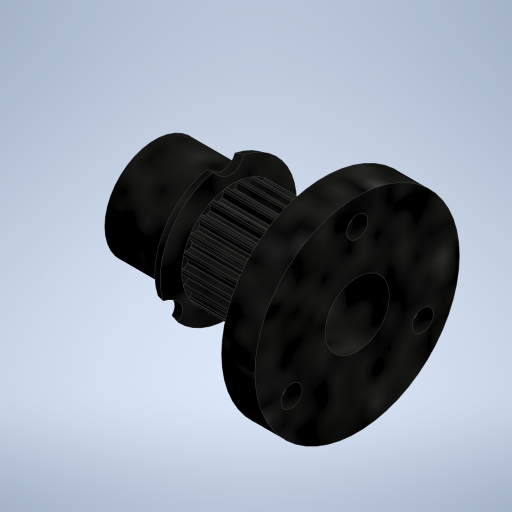
# Autodesk Inventor part: HTPA22S2M100-A-V4-Z6-J3.0_a
Saved by Autodesk Inventor 2024 (Build 280153000, 153)
## iProperties
Category: PARTsolutions
Company: MISUMI
Created: 2025-03-04
Part Number: HTPA22S2M100-A-V4-Z6-J3.0_a
Material: ABS プラスチック
Catalog Web Link: www.cadenas.de
Description: HTPA_ _S2M040, HTPA_ _S2M060, HTPA_ _S2M100, HTPB_ _S2M040, HTPB_ _S2M060, HTPB_ _S2M100, HTPK_ _S2M040, HTPK_ _S2M060, HTPK_ _S2M100, HTPN_ _S2M040, HTPN_ _S2M060, HTPN_ _S2M100, HTPT_ _S2M040, HTPT_ _S2M060, HTPM_ _S2M040, HTPM_ _S2M060, HTPP_ _S2M040, HTPP_ _S2M060, HTPS_ _S2M040, HTPS_ _S2M060, HTPS_ _S2M100_a-High Torque Timing Pulleys S2M Type
Vendor: MISUMI
Document SubType Name: Modeling
Designer: psAdmin
Manufacturer: MISUMI
Mass: 1.84697 g
Surface Area: 17.6348 cm^2
Volume: 1.84697 cm^3
Density: 1.06 g/cm^3
Appearance: 滑らか - 黒
PSOL_IDENT_0: {$CADENAS_DATA/23d-libs/misumi/metric/51_timing_pulleys/htpm_s2m/htpa_s2m.prj},750 {VTYP=3D},{NB=HTP
PSOL_IDENT_1: A22S2M100-A-V4-Z6-J3.0_a},{LINA=HTPA22S2M100-A-V4-Z6-J3.0},{NN=HTPA_ _S2M040, HTPA_ _S2M060, HTPA_ _
PSOL_IDENT_2: S2M100, HTPB_ _S2M040, HTPB_ _S2M060, HTPB_ _S2M100, HTPK_ _S2M040, HTPK_ _S2M060, HTPK_ _S2M100, HT
PSOL_IDENT_3: PN_ _S2M040, HTPN_ _S2M060, HTPN_ _S2M100, HTPT_ _S2M040, HTPT_ _S2M060, HTPM_ _S2M040, HTPM_ _S2M06
PSOL_IDENT_4: 0, HTPP_ _S2M040, HTPP_ _S2M060, HTPS_ _S2M040, HTPS_ _S2M060, HTPS_ _S2M100_a},{DATE=29.05.2023 09:
PSOL_IDENT_5: 16:33},{GEOMDATE=11.01.2023 01:57:31},{VERSION=},{LINEID=70},{WBVAR=MATP,ST,TNW,PS,SBS,DD,Z,J,Q,R,S,
PSOL_IDENT_6: T,ALT1,ALT2,M,QSC,QFC,QTC,ALT3,K,KSC,KFC,KTC,ALT4,ZM,ZSC,ZFC,ZTC,ALT5,ALT6,ALT7,FC,ALT8,SRG,ALT9,BTC
PSOL_IDENT_7: ,TL,ALT10,TPC,ALT11,BC,ALT12,SLH,ALT13,BN},{WBNUMERIC=DD,Z,J,Q,R,S,T,QSC,QFC,QTC,K,KSC,KFC,KTC,ZSC,Z
PSOL_IDENT_8: FC,ZTC,FC,SRG,BTC,TL,BC,SLH,BN}  {NB=HTPA22S2M100-A-V4-Z6-J3.0_a},{LINA=HTPA22S2M100-A-V4-Z6-J3.0},{
PSOL_IDENT_9: KT=DUMMY},{PN=HTPA22S2M100-A-V4-Z6-J3.0},{TYPE=HTPA},{MATP=A2017},{MATPALG= 'A2017','Aluminum Alloy
PSOL_IDENT_10: 2000 series','S45CE','1045 Carbon Steel Equivalent','SUS304','304 Stainless Steel' },{ST=CA},{STALG=
PSOL_IDENT_11: 'CA' , 'Clear Anodize', 'BA','Black Anodize','HAT','Hard Clear Anodize' , 'ENP' , 'Electroless Nick
PSOL_IDENT_12: el Plating' },{NT=22},{TNW=S2M100},{TNWALG= 'S2M040', 'S2M060','S2M100' },{BW=10},{PS=A},{PSALG='A','
PSOL_IDENT_13: K'},{SBS=V},{SBSALG= 'H', 'Round Hole','V','Stepped Hole','Y','Both Ends Stepped Hole','WB','Double
PSOL_IDENT_14: Stepped Hole' },{SHSA= 'H', 'Round Hole','V','Stepped Hole','Y','Both Ends Stepped Hole','WB','Doubl
PSOL_IDENT_15: e Stepped Hole' },{SHSB='H','Round Hole','P','Round Hole + Tap','N','New JIS Keywayed Bore + Tap (St
PSOL_IDENT_16: andard)','NK','New JIS Keywayed Bore + Tap (width 4.0mm, height 1.8mm)','C','Old JIS Keywayed Bore +
PSOL_IDENT_17: Tap','V','Stepped Hole','F','Stepped Hole (Counterbore holes on the boss side)' },{SHSK='H','Round
PSOL_IDENT_18: Hole','P','Round Hole + Tap'},{SBSPN=-V4-Z6-J3.0},{DD=4.00},{DDALG=[3:4/1],4.5,[5:5/1]},{DDHA=[3:4/1
PSOL_IDENT_19: ],4.5,[5:6/1],6.35,[7:8/1]},{DDHBK=0},{DDPA=0},{DDPBK=0},{DDNA=[8:8/1]},{DDNBK=0},{DDNK=0},{DDCA=0},
PSOL_IDENT_20: {DDCBK=0},{DDVA=[3:4/1],4.5,[5:5/1]},{DDVF=0},{DDY=[3:5/1]},{DDWB=[3:3/1]},{Z=6},{ZALG=[6:7/1]},{ZQR
PSOL_IDENT_21: MIN=6},{ZAMAX=7},{ZBMAX=0},{DDZ=6},{J=3.0},{JALG=[2:13/0.1]},{JMAX=13},{JMIN=2},{JPN=-J3.0},{QRMAX=7
PSOL_IDENT_22: },{QRMIN=6},{WBRMAX=-2.00},{WBQMIN=8},{Q=0},{QALG=[0]},{QPN=},{R=0},{RALG=[0]},{S=0.0},{SALG=[0]},{S
PSOL_IDENT_23: PN=},{SMAX=9},{T=0.0},{TALG=[0]},{TPN=},{TMAX=12},{A=11},{W=15},{L=0},{PD=14.01},{OD=13.50},{D=0},{D
PSOL_IDENT_24: ALG=18},{DE=11},{F=18},{E=11},{BBK=0.000},{TTK=0.0},{TT=1},{WL=15.000},{ALT1=},{ALT1ALG='','Not appl
PSOL_IDENT_25: icable'},{ANG=114.545},{ALT1PN=},{ALT2=},{ALT2ALG= '','Not applicable' },{M=N/A},{MALG= 'N/A' },{MFT
PSOL_IDENT_26: ALG= 'N/A' },{MSALG= 'N/A' },{M3D=0.000},{KDML=0},{ML=0},{MUL=0},{PITCH=0},{QSC=0.0},{QSCALG=0},{QFC=
PSOL_IDENT_27: 0.0},{QFCALG=0},{QTC=0.0},{QTCALG=0},{QPCDMIN=0},{QPCDMINALG=0},{QPCDMAX=7},{ALT2PN=},{ALT3=},{ALT3A
PSOL_IDENT_28: LG= '','Not applicable' },{K=0.0},{KALG=0},{KMIN=4},{KFTMAX=0.0},{KSMAX=0.0},{KSC=0.0},{KSCALG=0},{K
PSOL_IDENT_29: FC=0.0},{KFCALG=0},{KTC=0.0},{KTCALG=0},{KPCDMIN=10},{KPCDMINALG=10},{KPCDMAX=7},{KSCMIN=10.0},{KSCM
PSOL_IDENT_30: INALG=10},{ALT3PN=},{ALT4=},{ALT4ALG= '','Not applicable' },{ALT4MIN=16.5},{ALT4MAX=0.5},{ZM=N/A},{Z
PSOL_IDENT_31: MALG= 'N/A' },{ZMSALG= 'N/A' },{ZMFTALG= 'N/A' },{ZMDD1=0.0},{ZMDD2=0.0},{ZMHH=0.0},{ZSC=0.0},{ZSCAL
PSOL_IDENT_32: G=[0]},{ZFC=0.0},{ZFCALG=[0]},{ZTC=0.0},{ZTCALG=[0]},{ZPCDMIN=0},{ZPCDMINALG=0},{ZPCDMAX=7},{ALT4PN=
PSOL_IDENT_33: },{ALT5=},{ALT5ALG= '','Flange Attached','NFC','with NFC (Flange not Attached)' },{ALT5PN=},{ALT6=},
PSOL_IDENT_34: {ALT6ALG= '','w/o Flange Attached on One Side Only','RFC','with RFC (Flange Attached on The Boss Sid
PSOL_IDENT_35: e Only)','LFC','with LFC (Flange Attached on The Opposite Side Only)' },{ALT6PN=},{ALT7=},{ALT7ALG= ''
PSOL_IDENT_36: ,'w/o FC (Flange Cut)','FC','with FC (Flange Cut)' },{FC=0.0},{FCALG=0},{FCMIN=14.5},{FCMAX=16.0},{A
PSOL_IDENT_37: LT7PN=},{ALT8=},{ALT8ALG= '','Not applicable' },{ALT8ALGALG=7},{ALT8DD2=0},{ALT8MM=0},{ALT8NN=0},{QC=
PSOL_IDENT_38: 0},{KC=0},{ZC=0},{SRG=0.0},{SRGALG=[0]},{SRGMAX=0},{DD2=0.0},{MM=0.00},{NN=0.00},{ALT8PN=},{ALT9ALG=
PSOL_IDENT_39: '','Not applicable' },{ALT9=},{BTC9=6},{TL9=1},{BTC=0},{BTCALG=[0]},{TL=0.0},{TLALG=[0]},{TLMIN=1.0
PSOL_IDENT_40: },{TLMAX=-15.5},{BTCL=0},{BTCD=0},{BTCDALG=11.000},{ALT9PN=},{WLBCTL=15},{ALT10=},{ALT10ALG= '','Not
PSOL_IDENT_41: applicable' },{TPC=N/A},{TPCALG= 'N/A' },{TPCM=3},{ALT10PN=},{ALT11=},{ALT11ALG= '','Not applicable'
PSOL_IDENT_42: },{BC=0.0},{BCALG=0},{BCMIN=3},{BCMAX=-15.5},{BCPLANE=7.5},{M1WBC=7.5},{ALT11PN=},{ALT12=},{ALT12AL
PSOL_IDENT_43: G= '','Not applicable' },{SLH=0},{SLHALG=[0]},{ALT12PN=},{ALT13=},{ALT13ALG= '', 'Not applicable' },
PSOL_IDENT_44: {BN=0.0},{BNALG=0},{BNMIN=-14.5},{BNMAX=-5},{ALT13PN=},{AC=-},{M1=3},{M1L=3},{TAP=0.000},{KYY=2},{KT
PSOL_IDENT_45: T=4.75},{PLANE=15},{CD=0},{SRGCUT=1}
NB: HTPA22S2M100-A-V4-Z6-J3.0_a
NN: HTPA_ _S2M040, HTPA_ _S2M060, HTPA_ _S2M100, HTPB_ _S2M040, HTPB_ _S2M060, HTPB_ _S2M100, HTPK_ _S2M040, HTPK_ _S2M060, HTPK_ _S2M100, HTPN_ _S2M040, HTPN_ _S2M060, HTPN_ _S2M100, HTPT_ _S2M040, HTPT_ _S2M060, HTPM_ _S2M040, HTPM_ _S2M060, HTPP_ _S2M040, HTPP_ _S2M060, HTPS_ _S2M040, HTPS_ _S2M060, HTPS_ _S2M100_a
NT: 22
NBSYN: $PN._a
LINA: HTPA22S2M100-A-V4-Z6-J3.0
CATALOG: Misumi
PN: HTPA22S2M100-A-V4-Z6-J3.0
MATP: Aluminum Alloy 2000 series
ST: Clear Anodize
TNW: S2M100
BW: 10
PS: A
SBS: Stepped Hole
DD: 4
Z: 6
J: 3
Q: 0
R: 0
S: 0
T: 0
A: 11
W: 15
L: 0
PD: 14.01
OD: 13.5
D: 0
F: 18
ALT1: Not applicable
ALT2: Not applicable
M: N/A
QSC: 0
QFC: 0
QTC: 0
ALT3: Not applicable
K: 0
KSC: 0
KFC: 0
KTC: 0
ALT4: Not applicable
ZM: N/A
ZSC: 0
ZFC: 0
ZTC: 0
ALT5: Flange Attached
ALT6: w/o Flange Attached on One Side Only
ALT7: w/o FC (Flange Cut)
FC: 0
ALT8: Not applicable
SRG: 0
ALT9: Not applicable
BTC: 0
TL: 0
ALT10: Not applicable
TPC: N/A
ALT11: Not applicable
BC: 0
ALT12: Not applicable
SLH: 0
ALT13: Not applicable
BN: 0
AC: -
SUPPLIER: MISUMI
ARTICLENO: HTPA22S2M100-A-V4-Z6-J3.0_a
BOMINFO: HTPA22S2M100-A-V4-Z6-J3.0
CREATOR: CADENAS GmbH
Title: HTPA22S2M100-A-V4-Z6-J3.0
Author: Cadenas PARTsolutions
Comments: High Torque Timing Pulleys S2M Type
Autodesk Inventor part; units mm, degrees
sketch "_____1" plane through (0, 0, 0) normal (0, 0, 1) x (1, 0, 0)
  line L0 (15, 0) -> (0, 0)
  line L1 (0, 0) -> (0, 5.5)
  line L2 (0, 5.5) -> (1, 5.5)
  line L3 (1, 5.5) -> (1, 6.618348)
  line L4 (1, 6.618348) -> (0.431188, 8.741181)
  line L5 (0.431188, 8.741181) -> (1.397114, 9)
  line L6 (1.397114, 9) -> (2, 6.75)
  line L7 (2, 6.75) -> (13, 6.75)
  line L8 (13, 6.75) -> (13.602886, 9)
  line L9 (13.602886, 9) -> (14.568812, 8.741181)
  line L10 (14.568812, 8.741181) -> (14, 6.618348)
  line L11 (14, 6.618348) -> (14, 5.5)
  line L12 (14, 5.5) -> (15, 5.5)
  line L13 (15, 5.5) -> (15, 0)
  line L14 (15, 0) -> (0, 0)
  constraints: 30 end point
revolve "Revolution1" add sketch "_____1" angle 360 about axis through (15, 0, 0) along (1, 0, 0)
sketch "Sketch2" plane through (15, 0, 0) normal (1, 0, 0) x (0, 0, -1)
  point P0 (0, 0)
hole "Hole1" at (15, 0, 0) direction (-1, 0, 0) diameter 4 depth 15
sketch "_____6" plane through (2, 0, 0) normal (1, 0, 0) x (0, 0, -1)
  circle A0 centre (0, 0) radius 13.5
  arc A1 (-6.75, 0) -> (-6.748413, -0.146363) centre (0, 0) ccw
  arc A2 (-6.748413, -0.146363) -> (-6.590165, -0.329578) centre (-6.558458, -0.142243) ccw
  arc A3 (-5.990625, -0.595734) -> (-6.590165, -0.329578) centre (-6.81128, -1.635998) ccw
  arc A4 (-5.953176, -0.663173) -> (-5.990625, -0.595734) centre (-6.052561, -0.674244) ccw
  arc A5 (-5.953176, -0.663173) -> (-5.898868, -1.040894) centre (0, 0) ccw
  arc A6 (-5.9158, -1.116152) -> (-5.898868, -1.040894) centre (-5.997346, -1.058271) ccw
  arc A7 (-6.41607, -1.540436) -> (-5.9158, -1.116152) centre (-6.996289, -0.34923) ccw
  arc A8 (-6.41607, -1.540436) -> (-6.51629, -1.760814) centre (-6.332868, -1.71125) ccw
  arc A9 (-6.51629, -1.760814) -> (-6.476578, -1.901695) centre (0, 0) ccw
  arc A10 (-6.476578, -1.901695) -> (-6.43382, -2.041681) centre (0, 0) ccw
  arc A11 (-6.43382, -2.041681) -> (-6.230364, -2.172892) centre (-6.25272, -1.984212) ccw
  arc A12 (-5.580125, -2.259357) -> (-6.230364, -2.172892) centre (-6.074461, -3.488688) ccw
  arc A13 (-5.525193, -2.313513) -> (-5.580125, -2.259357) centre (-5.617433, -2.352136) ccw
  arc A14 (-5.525193, -2.313513) -> (-5.366669, -2.660633) centre (0, 0) ccw
  arc A15 (-5.361712, -2.737613) -> (-5.366669, -2.660633) centre (-5.456262, -2.705051) ccw
  arc A16 (-5.722183, -3.285653) -> (-5.361712, -2.737613) centre (-6.614501, -2.306167) ccw
  arc A17 (-5.722183, -3.285653) -> (-5.756256, -3.52534) centre (-5.594228, -3.426108) ccw
  arc A18 (-5.756256, -3.52534) -> (-5.678461, -3.649326) centre (0, 0) ccw
  arc A19 (-5.678461, -3.649326) -> (-5.597997, -3.771595) centre (0, 0) ccw
  arc A20 (-5.597997, -3.771595) -> (-5.365816, -3.840171) centre (-5.440423, -3.665432) ccw
  arc A21 (-4.717556, -3.73994) -> (-5.365816, -3.840171) centre (-4.845526, -5.058745) ccw
  arc A22 (-4.649592, -3.776427) -> (-4.717556, -3.73994) centre (-4.727214, -3.839472) ccw
  arc A23 (-4.649592, -3.776427) -> (-4.399694, -4.064824) centre (0, 0) ccw
  arc A24 (-4.373251, -4.137289) -> (-4.399694, -4.064824) centre (-4.473144, -4.132684) ccw
  arc A25 (-4.564719, -4.764686) -> (-4.373251, -4.137289) centre (-5.696845, -4.076271) ccw
  arc A26 (-4.564719, -4.764686) -> (-4.529884, -5.004263) centre (-4.402376, -4.863402) ccw
  arc A27 (-4.529884, -5.004263) -> (-4.42031, -5.10131) centre (0, 0) ccw
  arc A28 (-4.42031, -5.10131) -> (-4.308657, -5.195957) centre (0, 0) ccw
  arc A29 (-4.308657, -5.195957) -> (-4.066561, -5.196342) centre (-4.187377, -5.049701) ccw
  arc A30 (-3.472799, -4.917535) -> (-4.066561, -5.196342) centre (-3.224035, -6.218973) ccw
  arc A31 (-3.397308, -4.933396) -> (-3.472799, -4.917535) centre (-3.454025, -5.015757) ccw
  arc A32 (-3.397308, -4.933396) -> (-3.076282, -5.139707) centre (0, 0) ccw
  arc A33 (-3.030494, -5.201787) -> (-3.076282, -5.139707) centre (-3.127639, -5.225512) ccw
  arc A34 (-3.037448, -5.857713) -> (-3.030494, -5.201787) centre (-4.317664, -5.51614) ccw
  arc A35 (-3.037448, -5.857713) -> (-2.936528, -6.077771) centre (-2.85387, -5.906693) ccw
  arc A36 (-2.936528, -6.077771) -> (-2.804051, -6.140016) centre (0, 0) ccw
  arc A37 (-2.804051, -6.140016) -> (-2.670256, -6.199374) centre (0, 0) ccw
  arc A38 (-2.670256, -6.199374) -> (-2.437858, -6.131537) centre (-2.595093, -6.024873) ccw
  arc A39 (-1.946697, -5.696741) -> (-2.437858, -6.131537) centre (-1.341352, -6.875376) ccw
  arc A40 (-1.869795, -5.690691) -> (-1.946697, -5.696741) centre (-1.90101, -5.785694) ccw
  arc A41 (-1.869795, -5.690691) -> (-1.503648, -5.798202) centre (0, 0) ccw
  arc A42 (-1.442225, -5.844867) -> (-1.503648, -5.798202) centre (-1.528751, -5.895) ccw
  arc A43 (-1.264102, -6.476183) -> (-1.442225, -5.844867) centre (-2.588692, -6.509124) ccw
  arc A44 (-1.264102, -6.476183) -> (-1.105272, -6.658894) centre (-1.074161, -6.471459) ccw
  arc A45 (-1.105272, -6.658894) -> (-0.960625, -6.681295) centre (0, 0) ccw
  arc A46 (-0.960625, -6.681295) -> (-0.815527, -6.700553) centre (0, 0) ccw
  arc A47 (-0.815527, -6.700553) -> (-0.611655, -6.56999) centre (-0.792571, -6.511945) ccw
  arc A48 (-0.262885, -6.014431) -> (-0.611655, -6.56999) centre (0.65, -6.974778) ccw
  arc A49 (-0.190802, -5.98696) -> (-0.262885, -6.014431) centre (-0.193988, -6.08691) ccw
  arc A50 (-0.190802, -5.98696) -> (0.190802, -5.98696) centre (0, 0) ccw
  arc A51 (0.262885, -6.014431) -> (0.190802, -5.98696) centre (0.193988, -6.08691) ccw
  arc A52 (0.611655, -6.56999) -> (0.262885, -6.014431) centre (-0.65, -6.974778) ccw
  arc A53 (0.611655, -6.56999) -> (0.815527, -6.700553) centre (0.792571, -6.511945) ccw
  arc A54 (0.815527, -6.700553) -> (0.960625, -6.681295) centre (0, 0) ccw
  arc A55 (0.960625, -6.681295) -> (1.105272, -6.658894) centre (0, 0) ccw
  arc A56 (1.105272, -6.658894) -> (1.264102, -6.476183) centre (1.074161, -6.471459) ccw
  arc A57 (1.442225, -5.844867) -> (1.264102, -6.476183) centre (2.588692, -6.509124) ccw
  arc A58 (1.503648, -5.798202) -> (1.442225, -5.844867) centre (1.528751, -5.895) ccw
  arc A59 (1.503648, -5.798202) -> (1.869795, -5.690691) centre (0, 0) ccw
  arc A60 (1.946697, -5.696741) -> (1.869795, -5.690691) centre (1.90101, -5.785694) ccw
  arc A61 (2.437858, -6.131536) -> (1.946697, -5.696741) centre (1.341352, -6.875376) ccw
  arc A62 (2.437858, -6.131536) -> (2.670256, -6.199374) centre (2.595093, -6.024873) ccw
  arc A63 (2.670256, -6.199374) -> (2.804051, -6.140016) centre (0, 0) ccw
  arc A64 (2.804051, -6.140016) -> (2.936528, -6.077771) centre (0, 0) ccw
  arc A65 (2.936528, -6.077771) -> (3.037448, -5.857713) centre (2.85387, -5.906693) ccw
  arc A66 (3.030494, -5.201787) -> (3.037448, -5.857713) centre (4.317664, -5.51614) ccw
  arc A67 (3.076282, -5.139707) -> (3.030494, -5.201787) centre (3.127639, -5.225512) ccw
  arc A68 (3.076282, -5.139707) -> (3.397308, -4.933396) centre (0, 0) ccw
  arc A69 (3.472799, -4.917535) -> (3.397308, -4.933396) centre (3.454025, -5.015757) ccw
  arc A70 (4.066561, -5.196342) -> (3.472799, -4.917535) centre (3.224035, -6.218973) ccw
  arc A71 (4.066561, -5.196342) -> (4.308657, -5.195957) centre (4.187377, -5.049701) ccw
  arc A72 (4.308657, -5.195957) -> (4.42031, -5.10131) centre (0, 0) ccw
  arc A73 (4.42031, -5.10131) -> (4.529884, -5.004263) centre (0, 0) ccw
  arc A74 (4.529884, -5.004263) -> (4.564719, -4.764686) centre (4.402376, -4.863402) ccw
  arc A75 (4.373251, -4.137289) -> (4.564719, -4.764686) centre (5.696845, -4.076271) ccw
  arc A76 (4.399694, -4.064824) -> (4.373251, -4.137289) centre (4.473144, -4.132684) ccw
  arc A77 (4.399694, -4.064824) -> (4.649592, -3.776427) centre (0, 0) ccw
  arc A78 (4.717556, -3.73994) -> (4.649592, -3.776427) centre (4.727214, -3.839472) ccw
  arc A79 (5.365816, -3.840171) -> (4.717556, -3.73994) centre (4.845526, -5.058745) ccw
  arc A80 (5.365816, -3.840171) -> (5.597997, -3.771595) centre (5.440423, -3.665432) ccw
  arc A81 (5.597997, -3.771595) -> (5.678461, -3.649326) centre (0, 0) ccw
  arc A82 (5.678461, -3.649326) -> (5.756256, -3.52534) centre (0, 0) ccw
  arc A83 (5.756256, -3.52534) -> (5.722183, -3.285653) centre (5.594228, -3.426108) ccw
  arc A84 (5.361712, -2.737613) -> (5.722183, -3.285653) centre (6.614501, -2.306167) ccw
  arc A85 (5.366669, -2.660633) -> (5.361712, -2.737613) centre (5.456262, -2.705051) ccw
  arc A86 (5.366669, -2.660633) -> (5.525193, -2.313513) centre (0, 0) ccw
  arc A87 (5.580125, -2.259357) -> (5.525193, -2.313513) centre (5.617433, -2.352136) ccw
  arc A88 (6.230364, -2.172892) -> (5.580125, -2.259357) centre (6.074461, -3.488688) ccw
  arc A89 (6.230364, -2.172892) -> (6.43382, -2.041681) centre (6.25272, -1.984212) ccw
  arc A90 (6.43382, -2.041681) -> (6.476578, -1.901695) centre (0, 0) ccw
  arc A91 (6.476578, -1.901695) -> (6.51629, -1.760814) centre (0, 0) ccw
  arc A92 (6.51629, -1.760814) -> (6.41607, -1.540436) centre (6.332868, -1.71125) ccw
  arc A93 (5.9158, -1.116152) -> (6.41607, -1.540436) centre (6.996289, -0.34923) ccw
  arc A94 (5.898868, -1.040894) -> (5.9158, -1.116152) centre (5.997346, -1.058271) ccw
  arc A95 (5.898868, -1.040894) -> (5.953176, -0.663173) centre (0, 0) ccw
  arc A96 (5.990625, -0.595734) -> (5.953176, -0.663173) centre (6.052561, -0.674244) ccw
  arc A97 (6.590165, -0.329578) -> (5.990625, -0.595734) centre (6.81128, -1.635998) ccw
  arc A98 (6.590165, -0.329578) -> (6.748413, -0.146363) centre (6.558458, -0.142243) ccw
  arc A99 (6.748413, -0.146363) -> (6.75, 0) centre (0, 0) ccw
  arc A100 (6.75, 0) -> (6.748413, 0.146363) centre (0, 0) ccw
  arc A101 (6.748413, 0.146363) -> (6.590165, 0.329578) centre (6.558458, 0.142243) ccw
  arc A102 (5.990625, 0.595734) -> (6.590165, 0.329578) centre (6.81128, 1.635998) ccw
  arc A103 (5.953176, 0.663173) -> (5.990625, 0.595734) centre (6.052561, 0.674244) ccw
  arc A104 (5.953176, 0.663173) -> (5.898868, 1.040894) centre (0, 0) ccw
  arc A105 (5.9158, 1.116152) -> (5.898868, 1.040894) centre (5.997346, 1.058271) ccw
  arc A106 (6.41607, 1.540436) -> (5.9158, 1.116152) centre (6.996289, 0.34923) ccw
  arc A107 (6.41607, 1.540436) -> (6.51629, 1.760814) centre (6.332868, 1.71125) ccw
  arc A108 (6.51629, 1.760814) -> (6.476578, 1.901695) centre (0, 0) ccw
  arc A109 (6.476578, 1.901695) -> (6.43382, 2.041681) centre (0, 0) ccw
  arc A110 (6.43382, 2.041681) -> (6.230364, 2.172892) centre (6.25272, 1.984212) ccw
  arc A111 (5.580125, 2.259357) -> (6.230364, 2.172892) centre (6.074461, 3.488688) ccw
  arc A112 (5.525193, 2.313513) -> (5.580125, 2.259357) centre (5.617433, 2.352136) ccw
  arc A113 (5.525193, 2.313513) -> (5.366669, 2.660633) centre (0, 0) ccw
  arc A114 (5.361712, 2.737613) -> (5.366669, 2.660633) centre (5.456262, 2.705051) ccw
  arc A115 (5.722183, 3.285653) -> (5.361712, 2.737613) centre (6.614501, 2.306167) ccw
  arc A116 (5.722183, 3.285653) -> (5.756256, 3.52534) centre (5.594228, 3.426108) ccw
  arc A117 (5.756256, 3.52534) -> (5.678461, 3.649326) centre (0, 0) ccw
  arc A118 (5.678461, 3.649326) -> (5.597997, 3.771595) centre (0, 0) ccw
  arc A119 (5.597997, 3.771595) -> (5.365816, 3.840171) centre (5.440423, 3.665432) ccw
  arc A120 (4.717556, 3.73994) -> (5.365816, 3.840171) centre (4.845526, 5.058745) ccw
  arc A121 (4.649592, 3.776426) -> (4.717556, 3.73994) centre (4.727214, 3.839472) ccw
  arc A122 (4.649592, 3.776426) -> (4.399694, 4.064824) centre (0, 0) ccw
  arc A123 (4.373251, 4.137289) -> (4.399694, 4.064824) centre (4.473144, 4.132684) ccw
  arc A124 (4.564719, 4.764686) -> (4.373251, 4.137289) centre (5.696845, 4.076271) ccw
  arc A125 (4.564719, 4.764686) -> (4.529884, 5.004263) centre (4.402376, 4.863402) ccw
  arc A126 (4.529884, 5.004263) -> (4.42031, 5.10131) centre (0, 0) ccw
  arc A127 (4.42031, 5.10131) -> (4.308657, 5.195957) centre (0, 0) ccw
  arc A128 (4.308657, 5.195957) -> (4.066561, 5.196342) centre (4.187377, 5.049701) ccw
  arc A129 (3.472799, 4.917535) -> (4.066561, 5.196342) centre (3.224035, 6.218973) ccw
  arc A130 (3.397308, 4.933396) -> (3.472799, 4.917535) centre (3.454025, 5.015757) ccw
  arc A131 (3.397308, 4.933396) -> (3.076282, 5.139707) centre (0, 0) ccw
  arc A132 (3.030494, 5.201787) -> (3.076282, 5.139707) centre (3.127639, 5.225512) ccw
  arc A133 (3.037448, 5.857713) -> (3.030494, 5.201787) centre (4.317664, 5.51614) ccw
  arc A134 (3.037448, 5.857713) -> (2.936528, 6.077771) centre (2.85387, 5.906693) ccw
  arc A135 (2.936528, 6.077771) -> (2.804051, 6.140016) centre (0, 0) ccw
  arc A136 (2.804051, 6.140016) -> (2.670256, 6.199374) centre (0, 0) ccw
  arc A137 (2.670256, 6.199374) -> (2.437858, 6.131537) centre (2.595093, 6.024873) ccw
  arc A138 (1.946697, 5.696741) -> (2.437858, 6.131537) centre (1.341352, 6.875376) ccw
  arc A139 (1.869795, 5.690691) -> (1.946697, 5.696741) centre (1.90101, 5.785694) ccw
  arc A140 (1.869795, 5.690691) -> (1.503648, 5.798202) centre (0, 0) ccw
  arc A141 (1.442225, 5.844867) -> (1.503648, 5.798202) centre (1.528751, 5.895) ccw
  arc A142 (1.264102, 6.476183) -> (1.442225, 5.844867) centre (2.588692, 6.509124) ccw
  arc A143 (1.264102, 6.476183) -> (1.105272, 6.658894) centre (1.074161, 6.471459) ccw
  arc A144 (1.105272, 6.658894) -> (0.960625, 6.681295) centre (0, 0) ccw
  arc A145 (0.960625, 6.681295) -> (0.815526, 6.700553) centre (0, 0) ccw
  arc A146 (0.815526, 6.700553) -> (0.611655, 6.56999) centre (0.792571, 6.511945) ccw
  arc A147 (0.262885, 6.014431) -> (0.611655, 6.56999) centre (-0.65, 6.974778) ccw
  arc A148 (0.190802, 5.98696) -> (0.262885, 6.014431) centre (0.193988, 6.08691) ccw
  arc A149 (0.190802, 5.98696) -> (-0.190802, 5.98696) centre (0, 0) ccw
  arc A150 (-0.262885, 6.014431) -> (-0.190802, 5.98696) centre (-0.193988, 6.08691) ccw
  arc A151 (-0.611654, 6.56999) -> (-0.262885, 6.014431) centre (0.65, 6.974778) ccw
  arc A152 (-0.611654, 6.56999) -> (-0.815527, 6.700553) centre (-0.792571, 6.511945) ccw
  arc A153 (-0.815527, 6.700553) -> (-0.960625, 6.681295) centre (0, 0) ccw
  arc A154 (-0.960625, 6.681295) -> (-1.105272, 6.658894) centre (0, 0) ccw
  arc A155 (-1.105272, 6.658894) -> (-1.264102, 6.476183) centre (-1.074161, 6.471459) ccw
  arc A156 (-1.442225, 5.844867) -> (-1.264102, 6.476183) centre (-2.588692, 6.509124) ccw
  arc A157 (-1.503648, 5.798202) -> (-1.442225, 5.844867) centre (-1.528751, 5.895) ccw
  arc A158 (-1.503648, 5.798202) -> (-1.869795, 5.690691) centre (0, 0) ccw
  arc A159 (-1.946697, 5.696741) -> (-1.869795, 5.690691) centre (-1.90101, 5.785694) ccw
  arc A160 (-2.437858, 6.131536) -> (-1.946697, 5.696741) centre (-1.341352, 6.875376) ccw
  arc A161 (-2.437858, 6.131536) -> (-2.670256, 6.199374) centre (-2.595093, 6.024873) ccw
  arc A162 (-2.670256, 6.199374) -> (-2.804051, 6.140016) centre (0, 0) ccw
  arc A163 (-2.804051, 6.140016) -> (-2.936528, 6.077771) centre (0, 0) ccw
  arc A164 (-2.936528, 6.077771) -> (-3.037448, 5.857713) centre (-2.85387, 5.906693) ccw
  arc A165 (-3.030494, 5.201787) -> (-3.037448, 5.857713) centre (-4.317664, 5.51614) ccw
  arc A166 (-3.076282, 5.139707) -> (-3.030494, 5.201787) centre (-3.127639, 5.225512) ccw
  arc A167 (-3.076282, 5.139707) -> (-3.397308, 4.933396) centre (0, 0) ccw
  arc A168 (-3.472799, 4.917535) -> (-3.397308, 4.933396) centre (-3.454025, 5.015757) ccw
  arc A169 (-4.066561, 5.196342) -> (-3.472799, 4.917535) centre (-3.224035, 6.218973) ccw
  arc A170 (-4.066561, 5.196342) -> (-4.308657, 5.195957) centre (-4.187377, 5.049701) ccw
  arc A171 (-4.308657, 5.195957) -> (-4.42031, 5.10131) centre (0, 0) ccw
  arc A172 (-4.42031, 5.10131) -> (-4.529884, 5.004263) centre (0, 0) ccw
  arc A173 (-4.529884, 5.004263) -> (-4.564719, 4.764686) centre (-4.402376, 4.863402) ccw
  arc A174 (-4.373251, 4.137289) -> (-4.564719, 4.764686) centre (-5.696845, 4.076271) ccw
  arc A175 (-4.399694, 4.064824) -> (-4.373251, 4.137289) centre (-4.473144, 4.132684) ccw
  arc A176 (-4.399694, 4.064824) -> (-4.649592, 3.776427) centre (0, 0) ccw
  arc A177 (-4.717556, 3.73994) -> (-4.649592, 3.776427) centre (-4.727214, 3.839472) ccw
  arc A178 (-5.365816, 3.840171) -> (-4.717556, 3.73994) centre (-4.845526, 5.058745) ccw
  arc A179 (-5.365816, 3.840171) -> (-5.597997, 3.771595) centre (-5.440423, 3.665432) ccw
  arc A180 (-5.597997, 3.771595) -> (-5.678461, 3.649326) centre (0, 0) ccw
  arc A181 (-5.678461, 3.649326) -> (-5.756256, 3.525339) centre (0, 0) ccw
  arc A182 (-5.756256, 3.525339) -> (-5.722183, 3.285653) centre (-5.594228, 3.426108) ccw
  arc A183 (-5.361712, 2.737613) -> (-5.722183, 3.285653) centre (-6.614501, 2.306167) ccw
  arc A184 (-5.366669, 2.660633) -> (-5.361712, 2.737613) centre (-5.456262, 2.705051) ccw
  arc A185 (-5.366669, 2.660633) -> (-5.525193, 2.313513) centre (0, 0) ccw
  arc A186 (-5.580125, 2.259357) -> (-5.525193, 2.313513) centre (-5.617433, 2.352136) ccw
  arc A187 (-6.230364, 2.172892) -> (-5.580125, 2.259357) centre (-6.074461, 3.488688) ccw
  arc A188 (-6.230364, 2.172892) -> (-6.43382, 2.041681) centre (-6.25272, 1.984212) ccw
  arc A189 (-6.43382, 2.041681) -> (-6.476578, 1.901695) centre (0, 0) ccw
  arc A190 (-6.476578, 1.901695) -> (-6.51629, 1.760814) centre (0, 0) ccw
  arc A191 (-6.51629, 1.760814) -> (-6.41607, 1.540436) centre (-6.332868, 1.71125) ccw
  arc A192 (-5.9158, 1.116152) -> (-6.41607, 1.540436) centre (-6.996289, 0.34923) ccw
  arc A193 (-5.898868, 1.040894) -> (-5.9158, 1.116152) centre (-5.997346, 1.058271) ccw
  arc A194 (-5.898868, 1.040894) -> (-5.953176, 0.663173) centre (0, 0) ccw
  arc A195 (-5.990625, 0.595734) -> (-5.953176, 0.663173) centre (-6.052561, 0.674244) ccw
  arc A196 (-6.590165, 0.329578) -> (-5.990625, 0.595734) centre (-6.81128, 1.635998) ccw
  arc A197 (-6.590165, 0.329578) -> (-6.748413, 0.146363) centre (-6.558458, 0.142243) ccw
  arc A198 (-6.748413, 0.146363) -> (-6.75, 0) centre (0, 0) ccw
  constraints: 396 point on circle, 199 centre point
extrude "Extrusion1" cut sketch "_____6" along normal blind 11
sketch "_____11" plane through (0, 0, 0) normal (0, 0, 1) x (1, 0, 0)
  line L0 (3, 0) -> (0, 0)
  line L1 (0, 0) -> (0, 3)
  line L2 (0, 3) -> (3, 3)
  line L3 (3, 3) -> (3, 0)
  line L4 (3, 0) -> (0, 0)
  constraints: 10 end point
revolve "Revolution2" cut sketch "_____11" angle 360 about axis through (3, 0, 0) along (1, 0, 0)
ref_plane "C1_XY" through (7.5, 0, 0) normal (1, 0, 0) x (0, 0, -1)
ref_plane "C1_YZ" through (7.5, 0, 0) normal (0, 0, -1) x (0, 1, 0)
ref_plane "C1_ZX" through (7.5, 0, 0) normal (0, 1, 0) x (1, 0, 0)
ref_plane "to_belt_XY" through (7.5, 0, 0) normal (-1, 0, 0) x (0, 0, -1)
ref_plane "to_belt_YZ" through (7.5, 0, 0) normal (0, 0, -1) x (0, -1, 0)
ref_plane "to_belt_ZX" through (7.5, 0, 0) normal (0, -1, 0) x (-1, 0, 0)
sketch "スケッチ5" plane through (15, 0, 0) normal (1, 0, 0) x (0, 0, -1)
  circle A0 centre (0, 0) radius 9
  constraints: 1 centre point, 1 coincident
extrude "押し出し2" cut sketch "スケッチ5" against normal blind 1
sketch "スケッチ6" plane through (14, 0, 0) normal (1, 0, 0) x (0, 0, -1)
  circle A0 centre (0, 0) radius 13.5
  dimension "d13" = 27
  constraints: 1 centre point, 1 coincident
  measures "d13" diameter of A0
extrude "押し出し3" add sketch "スケッチ6" along normal blind 3
sketch "スケッチ7" plane through (17, 0, 0) normal (1, 0, 0) x (0, 0, -1)
  circle A0 centre (0, 0) radius 10
  circle A1 centre (0, 10) radius 1
  circle A2 centre (-8.660254, -5) radius 1
  circle A3 centre (8.660254, -5) radius 1
  dimension "d16" = 20
  dimension "d17" = 2
  dimension "d20" = 360
  constraints: 3 centre point, 1 coincident, 1 vertical alignment, 9 other
  measures "d17" diameter of A1
extrude "押し出し4" cut sketch "スケッチ7" against normal blind 3 contours A1 A0 | A0 A1 | A3 A0 | A0 A3 | A2 A0 | A0 A2
sketch "スケッチ8" plane through (14, 0, 0) normal (-1, 0, 0) x (0, 0, 1)
  circle A0 centre (-8.660254, -5) radius 1
  circle A1 centre (-8.660254, -5) radius 2.35
  circle A2 centre (0, 10) radius 1
  circle A3 centre (0, 10) radius 2.35
  circle A4 centre (8.660254, -5) radius 1
  circle A5 centre (8.660254, -5) radius 2.35
  point P0 (0, 0)
  dimension "d24" = 4.7
  dimension "d25" = 4.7
  dimension "d26" = 4.7
  constraints: 3 centre point, 3 coincident
  measures "d24" diameter of A1
  measures "d25" diameter of A3
  measures "d26" diameter of A5
extrude "押し出し5" cut sketch "スケッチ8" along normal blind 2 and the other way blind 2.5
sketch "スケッチ9" plane through (17, 0, 0) normal (1, 0, 0) x (0, 0, -1)
  circle A0 centre (0, 0) radius 13.5
  constraints: 1 centre point, 1 coincident
extrude "押し出し6" add sketch "スケッチ9" along normal blind 0.9
sketch "スケッチ10" plane through (17, 10, 0) normal (-1, 0, 0) x (0, 0, 1)
  circle A0 centre (0, 0) radius 1
  circle A1 centre (8.660254, -15) radius 1
  circle A2 centre (8.660254, -15) radius 1
  circle A3 centre (-8.660254, -15) radius 1
  circle A4 centre (-8.660254, -15) radius 1
  point P0 (0, -10)
  constraints: 3 centre point, 2 coincident
extrude "押し出し7" cut sketch "スケッチ10" against normal blind 0.7
sketch "スケッチ11" plane through (16.5, -5, -8.660254) normal (-1, 0, 0) x (0, 0, 1)
  circle A0 centre (0, 0) radius 1.4
  circle A1 centre (8.660254, 15) radius 1
  circle A2 centre (8.660254, 15) radius 1.4
  circle A3 centre (17.320508, 0) radius 1
  circle A4 centre (17.320508, 0) radius 1.4
  point P0 (8.660254, 5)
  dimension "d35" = 2.8
  dimension "d36" = 2.8
  dimension "d37" = 2.8
  constraints: 3 centre point, 2 coincident
  measures "d35" diameter of A0
  measures "d36" diameter of A2
  measures "d37" diameter of A4
extrude "押し出し8" cut sketch "スケッチ11" against normal blind 10
sketch "スケッチ12" plane through (17.9, 10, 0) normal (1, 0, 0) x (0, 0, -1)
  circle A0 centre (0, 0) radius 1
  point P0 (0, -10)
  constraints: 1 centre point
extrude "押し出し9" cut sketch "スケッチ12" against normal blind 0.9
sketch "スケッチ13" plane through (17.9, -5, 8.660254) normal (1, 0, 0) x (0, 0, -1)
  circle A0 centre (0, 0) radius 1
  point P0 (8.660254, 5)
  constraints: 1 centre point
extrude "押し出し10" cut sketch "スケッチ13" against normal blind 0.9
sketch "スケッチ14" plane through (17.9, 0, 0) normal (1, 0, 0) x (0, 0, -1)
  circle A0 centre (0, 0) radius 13.5
  constraints: 1 centre point, 1 coincident
extrude "押し出し11" add sketch "スケッチ14" along normal blind 0.5
sketch "スケッチ15" plane through (17.9, 10, 0) normal (-1, 0, 0) x (0, 0, 1)
  circle A0 centre (0, 0) radius 1.4
  circle A1 centre (8.660254, -15) radius 1.4
  circle A2 centre (8.660254, -15) radius 1.4
  circle A3 centre (-8.660254, -15) radius 1.4
  circle A4 centre (-8.660254, -15) radius 1.4
  point P0 (0, -10)
  constraints: 3 centre point, 2 coincident
extrude "押し出し12" cut sketch "スケッチ15" against normal blind 0.5
sketch "スケッチ16" plane through (0, 0, 0) normal (-1, 0, 0) x (0, 0, 1)
  circle A0 centre (0, 0) radius 5.5
  constraints: 1 centre point, 1 coincident
extrude "押し出し13" add sketch "スケッチ16" along normal blind 8.3
sketch "スケッチ17" plane through (-8.3, 0, 0) normal (-1, 0, 0) x (0, 0, 1)
  circle A0 centre (0, 0) radius 2 projected
  circle A1 centre (0, 0) radius 2
  constraints: 1 centre point, 1 coincident
extrude "押し出し14" cut sketch "スケッチ17" against normal blind 30
sketch "スケッチ18" plane through (18.4, 0, 0) normal (1, 0, 0) x (0, 0, -1)
  circle A0 centre (8.660254, -5) radius 1.4
  circle A1 centre (8.660254, -5) radius 1.4
  circle A2 centre (-8.660254, -5) radius 1.4
  circle A3 centre (-8.660254, -5) radius 1.4
  circle A4 centre (0, 10) radius 1.4
  circle A5 centre (0, 10) radius 1.4
  point P0 (0, 0)
  constraints: 3 centre point, 3 coincident
extrude "押し出し15" cut sketch "スケッチ18" against normal blind 30
sketch "スケッチ19" plane through (18.4, 0, 0) normal (1, 0, 0) x (0, 0, -1)
  arc A0 (-7.267575, -4.857016) -> (7.267575, -4.857016) centre (0, 0) ccw
  circle A1 centre (0, 0) radius 4.25
  dimension "d54" = 8.5
  constraints: 1 centre point, 1 coincident
  measures "d54" diameter of A1
extrude "押し出し16" cut sketch "スケッチ19" against normal blind 8
sketch "スケッチ20" plane through (-8.3, 0, 0) normal (-1, 0, 0) x (0, 0, 1)
  circle A0 centre (0, 0) radius 3.5
  dimension "d57" = 7
  constraints: 1 centre point, 1 coincident
  measures "d57" diameter of A0
extrude "押し出し17" cut sketch "スケッチ20" against normal blind 8
sketch "スケッチ21" plane through (16.5, -5, -8.660254) normal (-1, 0, 0) x (0, 0, 1)
  circle A0 centre (0, 0) radius 1.4
  circle A1 centre (0, 0) radius 2.35
  arc A2 (10.603602, 13.678675) -> (6.716906, 13.678675) centre (8.660254, 15) ccw
  circle A3 centre (8.660254, 15) radius 2.35
  circle A4 centre (17.320508, 0) radius 2.35
  circle A5 centre (17.320508, 0) radius 2.35
  point P0 (8.660254, 5)
  point P1 (6.716906, 13.678675)
  point P2 (10.603602, 13.678675)
  constraints: 3 centre point, 3 coincident
extrude "押し出し18" cut sketch "スケッチ21" along normal blind 30
sketch "スケッチ22" plane through (-8.3, 0, 0) normal (-1, 0, 0) x (0, 0, 1)
  circle A0 centre (0, 0) radius 5.5
  constraints: 1 centre point, 1 coincident
extrude "押し出し19" cut sketch "スケッチ22" against normal blind 0.7
sketch "スケッチ23" plane through (1, 0, 0) normal (-1, 0, 0) x (0, 0, 1)
  circle A0 centre (0, 0) radius 6.618348
  arc A1 (5.597997, 3.771595) -> (4.529884, 5.004263) centre (0, 0) ccw
  circle A2 centre (0, 0) radius 3.5
  constraints: 2 centre point, 2 coincident
extrude "押し出し20" add sketch "スケッチ23" along normal blind 9.3
sketch "スケッチ24" plane through (10.4, 0, 0) normal (1, 0, 0) x (0, 0, -1)
  circle A0 centre (0, 0) radius 3.5
  dimension "d66" = 7
  constraints: 1 centre point, 1 coincident
  measures "d66" diameter of A0
extrude "押し出し21" cut sketch "スケッチ24" against normal blind 3
sketch "スケッチ25" plane through (-0.3, 0, 0) normal (-1, 0, 0) x (0, 0, 1)
  circle A0 centre (0, 0) radius 3.5
  circle A1 centre (0, 0) radius 2 projected
  circle A2 centre (0, 0) radius 2
  constraints: 2 centre point, 2 coincident
extrude "押し出し22" add sketch "スケッチ25" along normal blind 5
body "Solid1"
